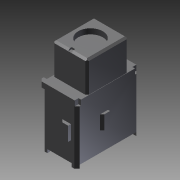
# Autodesk Inventor part: A1-toggle-body
Saved by Autodesk Inventor 2011 SP1 (Build 150282100, 282)
## iProperties
Created: 2013-12-24
Part Number: A1-toggle-body
Catalog Web Link: www.cadenas.de
Description: A Series - Process Sealed Subminiature Toggle -body-
Vendor: NKKSWITCHES
Document SubType Name: Modeling
Designer: PARTuser1
Manufacturer: NKKSWITCHES
Density: 1 g/cm^3
Category: PARTsolutions
Company: NKKSWITCHES
Title: A1-toggle-body
Author: Cadenas PARTsolutions
PSOL_IDENT_0: {$CADENAS_DATA\23d-libs\nkkswitches\toggle\a\parts\a_toggle_body.prj},218 {VTYP=3D},{NB=A1-toggle-bo
PSOL_IDENT_1: dy},{LINA=A1-toggle-body},{NN=A Series - Process Sealed Subminiature Toggle -body},{DATE=12.03.2009
PSOL_IDENT_2: 11:33:35},{GEOMDATE=26.02.2009 12:28:00},{VERSION=},{LINEID=10},{LINESUBID=-1},{WBVAR=PLS}  {NB=A1-t
PSOL_IDENT_3: oggle-body},{LINA=A1-toggle-body},{KT=DUMMY},{PN=A1},{SRS=A},{PLS=1}
CNS_NN: A Series - Process Sealed Subminiature Toggle -body
CNS_NB: A1-toggle-body
CNS_NBSYN: $PN.-toggle-body
CNS_LINA: A1-toggle-body
CNS_PN: A1
CNS_SRS: A
CNS_PLS: 1 - SPDT
SUPPLIER: NKKSWITCHES
ARTICLENO: A1-toggle-body
BOMINFO: A1-toggle-body
CREATOR: CADENAS GmbH
Autodesk Inventor part; units mm, degrees
sketch "Sketch_1" plane through (0, 0, 0) normal (0, 1, 0) x (-1, 0, 0)
  line L0 (2.54, -4.1148) -> (2.54, 4.1148)
  line L1 (2.54, 4.1148) -> (2.159, 4.4958)
  line L2 (2.159, 4.4958) -> (-2.159, 4.4958)
  line L3 (-2.159, 4.4958) -> (-2.54, 4.1148)
  line L4 (-2.54, 4.1148) -> (-2.54, -4.1148)
  line L5 (-2.54, -4.1148) -> (-2.159, -4.4958)
  line L6 (-2.159, -4.4958) -> (2.159, -4.4958)
  line L7 (2.159, -4.4958) -> (2.54, -4.1148)
  constraints: 16 end point
extrude "Extrusion1" add sketch "Sketch_1" against normal blind 8.6106
sketch "Sketch_2" plane through (0, -8.6106, 0) normal (0, 1, 0) x (1, 0, 0)
  line L0 (-2.54, 3.7338) -> (-2.54, -3.7338)
  line L1 (-2.54, -3.7338) -> (-2.159, -3.7338)
  line L2 (-2.159, -3.7338) -> (-2.159, -4.1148)
  line L3 (-2.159, -4.1148) -> (-1.778, -4.1148)
  line L4 (-1.778, -4.1148) -> (-1.778, -4.4958)
  line L5 (-1.778, -4.4958) -> (1.778, -4.4958)
  line L6 (1.778, -4.4958) -> (1.778, -4.1148)
  line L7 (1.778, -4.1148) -> (2.54, -4.1148)
  line L8 (2.54, -4.1148) -> (2.54, 4.1148)
  line L9 (2.54, 4.1148) -> (1.778, 4.1148)
  line L10 (1.778, 4.1148) -> (1.778, 4.4958)
  line L11 (1.778, 4.4958) -> (-1.778, 4.4958)
  line L12 (-1.778, 4.4958) -> (-1.778, 4.1148)
  line L13 (-1.778, 4.1148) -> (-2.159, 4.1148)
  line L14 (-2.159, 4.1148) -> (-2.159, 3.7338)
  line L15 (-2.159, 3.7338) -> (-2.54, 3.7338)
  constraints: 32 end point
extrude "Extrusion2" cut sketch "Sketch_2" along normal blind 0.508
sketch "Sketch_21" plane through (0, -8.6106, 0) normal (0, 1, 0) x (1, 0, 0)
  line L0 (-2.159, -4.1148) -> (2.159, -4.1148)
  line L1 (2.159, -4.1148) -> (2.159, 4.1148)
  line L2 (2.159, 4.1148) -> (-2.159, 4.1148)
  line L3 (-2.159, 4.1148) -> (-2.159, -4.1148)
  constraints: 8 end point
extrude "Extrusion3" cut sketch "Sketch_21" along normal blind 0.9144
sketch "Sketch_3" plane through (0, 0, 0) normal (0, 1, 0) x (-1, 0, 0)
  line L0 (-2.1717, -3.9243) -> (-2.6162, -3.9243)
  line L1 (-2.6162, -3.9243) -> (-2.6162, 3.9243)
  line L2 (-2.6162, 3.9243) -> (-2.1717, 3.9243)
  line L3 (-2.1717, 3.9243) -> (-2.1717, 4.4958)
  line L4 (-2.1717, 4.4958) -> (-2.921, 4.4958)
  line L5 (-2.921, 4.4958) -> (-2.921, -4.4958)
  line L6 (-2.921, -4.4958) -> (-2.1717, -4.4958)
  line L7 (-2.1717, -4.4958) -> (-2.1717, -3.9243)
  constraints: 16 end point
extrude "Extrusion4" cut sketch "Sketch_3" against normal blind 0.762
sketch "Sketch_4" plane through (0, 0, 0) normal (0, 1, 0) x (-1, 0, 0)
  line L0 (2.9972, -3.81) -> (2.5019, -3.81)
  line L1 (2.5019, -3.81) -> (2.5019, 3.81)
  line L2 (2.5019, 3.81) -> (2.9972, 3.81)
  line L3 (2.9972, 3.81) -> (2.9972, 4.1148)
  line L4 (2.9972, 4.1148) -> (2.6162, 4.4958)
  line L5 (2.6162, 4.4958) -> (0.0762, 4.4958)
  line L6 (0.0762, 4.4958) -> (0.0762, -4.4958)
  line L7 (0.0762, -4.4958) -> (2.6162, -4.4958)
  line L8 (2.6162, -4.4958) -> (2.9972, -4.1148)
  line L9 (2.9972, -4.1148) -> (2.9972, -3.81)
  constraints: 20 end point
extrude "Extrusion5" add sketch "Sketch_4" against normal blind 0.762
sketch "Sketch_5" plane through (0, -3.241, 0) normal (0, 1, 0) x (1, 0, 0)
  line L0 (0.41, -4.4958) -> (0.8164, -4.9022)
  line L1 (0.8164, -4.9022) -> (1.651, -4.9022)
  line L2 (1.651, -4.9022) -> (1.651, -4.4958)
  line L3 (1.651, -4.4958) -> (0.41, -4.4958)
  constraints: 8 end point
extrude "Extrusion6" add sketch "Sketch_5" against normal blind 2.032
sketch "Sketch_6" plane through (0, -3.241, 0) normal (0, 1, 0) x (1, 0, 0)
  line L0 (0.41, 4.4958) -> (1.651, 4.4958)
  line L1 (1.651, 4.4958) -> (1.651, 4.9022)
  line L2 (1.651, 4.9022) -> (0.8164, 4.9022)
  line L3 (0.8164, 4.9022) -> (0.41, 4.4958)
  constraints: 8 end point
extrude "Extrusion7" add sketch "Sketch_6" against normal blind 2.032
sketch "Sketch_7" plane through (0, -3.241, 0) normal (0, 1, 0) x (1, 0, 0)
  line L0 (2.54, 0) -> (2.54, -1.1394)
  line L1 (2.54, -1.1394) -> (2.8448, -0.8346)
  line L2 (2.8448, -0.8346) -> (2.8448, 0)
  line L3 (2.8448, 0) -> (2.54, 0)
  constraints: 8 end point
extrude "Extrusion8" add sketch "Sketch_7" against normal blind 2.032
sketch "Sketch_8" plane through (0, 0, 0) normal (0, 1, 0) x (-1, 0, 0)
  line L0 (2.5019, -2.7432) -> (2.5019, 2.7432)
  line L1 (2.5019, 2.7432) -> (2.2479, 2.9972)
  line L2 (2.2479, 2.9972) -> (-2.2479, 2.9972)
  line L3 (-2.2479, 2.9972) -> (-2.5019, 2.7432)
  line L4 (-2.5019, 2.7432) -> (-2.5019, -2.7432)
  line L5 (-2.5019, -2.7432) -> (-2.2479, -2.9972)
  line L6 (-2.2479, -2.9972) -> (2.2479, -2.9972)
  line L7 (2.2479, -2.9972) -> (2.5019, -2.7432)
  constraints: 16 end point
extrude "Extrusion9" add sketch "Sketch_8" along normal blind 4.4958
sketch "Sketch_9" plane through (0, 0, 0) normal (1, 0, 0) x (0, 1, 0)
  line L0 (0, 3.2953) -> (0, 2.9972)
  line L1 (0, 2.9972) -> (4.2418, 2.9972)
  line L2 (4.2418, 2.9972) -> (4.4958, 2.7432)
  line L3 (4.4958, 2.7432) -> (4.4958, -2.7432)
  line L4 (4.4958, -2.7432) -> (4.2418, -2.9972)
  line L5 (4.2418, -2.9972) -> (0, -2.9972)
  line L6 (0, -2.9972) -> (0, -3.2953)
  line L7 (0, -3.2953) -> (4.5957, -3.2953)
  line L8 (4.5957, -3.2953) -> (4.5957, 3.2953)
  line L9 (4.5957, 3.2953) -> (0, 3.2953)
  constraints: 20 end point
extrude "Extrusion10" cut sketch "Sketch_9" along normal mid plane 5.0038
sketch "Sketch_10" plane through (0, 0, 0) normal (0, 0, 1) x (1, 0, 0)
  line L0 (-3.2953, 0) -> (-2.5019, 0)
  line L1 (-2.5019, 0) -> (-2.5019, 4.2418)
  line L2 (-2.5019, 4.2418) -> (-2.2479, 4.4958)
  line L3 (-2.2479, 4.4958) -> (2.2479, 4.4958)
  line L4 (2.2479, 4.4958) -> (2.5019, 4.2418)
  line L5 (2.5019, 4.2418) -> (2.5019, 0)
  line L6 (2.5019, 0) -> (3.2953, 0)
  line L7 (3.2953, 0) -> (3.2953, 4.5957)
  line L8 (3.2953, 4.5957) -> (-3.2953, 4.5957)
  line L9 (-3.2953, 4.5957) -> (-3.2953, 0)
  constraints: 20 end point
extrude "Extrusion11" cut sketch "Sketch_10" along normal mid plane 5.9944
sketch "Sketch12" plane through (0, 4.4958, 0) normal (0, 1, 0) x (1, 0, 0)
  point P0 (0, 0)
hole "Drilling 1" at (0, 4.4958, 0) direction (0, -1, 0) diameter 3.556 depth 0.762
sketch "Sketch_28" plane through (0, 4.4958, 0) normal (0, 1, 0) x (1, 0, 0)
  line L0 (-0.254, -2.4892) -> (-0.254, -2.9972)
  line L1 (-0.254, -2.9972) -> (0.254, -2.9972)
  line L2 (0.254, -2.9972) -> (0.254, -2.4892)
  line L3 (0.254, -2.4892) -> (-0.254, -2.4892)
  constraints: 8 end point
extrude "Extrusion12" cut sketch "Sketch_28" against normal blind 0.254
ref_plane "to_bracket_r_XY" through (-2.54, -4.3078, 0) normal (1, 0, 0) x (0, 0, -1)
ref_plane "to_bracket_r_YZ" through (-2.54, -4.3078, 0) normal (0, 0, -1) x (0, 1, 0)
ref_plane "to_bracket_r_ZX" through (-2.54, -4.3078, 0) normal (0, 1, 0) x (1, 0, 0)
ref_plane "to_bracket_r2_XY" through (-4.3942, -4.318, 0) normal (1, 0, 0) x (0, 0, -1)
ref_plane "to_bracket_r2_YZ" through (-4.3942, -4.318, 0) normal (0, 0, -1) x (0, 1, 0)
ref_plane "to_bracket_r2_ZX" through (-4.3942, -4.318, 0) normal (0, 1, 0) x (1, 0, 0)
ref_plane "to_bracket_s_XY" through (-2.54, -4.7015, 0) normal (1, 0, 0) x (0, 0, -1)
ref_plane "to_bracket_s_YZ" through (-2.54, -4.7015, 0) normal (0, 0, -1) x (0, 1, 0)
ref_plane "to_bracket_s_ZX" through (-2.54, -4.7015, 0) normal (0, 1, 0) x (1, 0, 0)
ref_plane "to_bracket_s2_XY" through (-4.3942, -4.7142, 0) normal (1, 0, 0) x (0, 0, -1)
ref_plane "to_bracket_s2_YZ" through (-4.3942, -4.7142, 0) normal (0, 0, -1) x (0, 1, 0)
ref_plane "to_bracket_s2_ZX" through (-4.3942, -4.7142, 0) normal (0, 1, 0) x (1, 0, 0)
ref_plane "to_bracket_v_XY" through (0, -4.1554, 4.3942) normal (0, 0, -1) x (1, 0, 0)
ref_plane "to_bracket_v_YZ" through (0, -4.1554, 4.3942) normal (1, 0, 0) x (0, -1, 0)
ref_plane "to_bracket_v_ZX" through (0, -4.1554, 4.3942) normal (0, -1, 0) x (0, 0, -1)
ref_plane "to_dummy_XY" through (0, 0, 0) normal (0, -1, 0) x (1, 0, 0)
ref_plane "to_dummy_YZ" through (0, 0, 0) normal (1, 0, 0) x (0, 0, 1)
ref_plane "to_dummy_ZX" through (0, 0, 0) normal (0, 0, 1) x (0, -1, 0)
ref_plane "to_terminal_XY" through (0, -7.3406, 0) normal (0, 1, 0) x (1, 0, 0)
ref_plane "to_terminal_YZ" through (0, -7.3406, 0) normal (1, 0, 0) x (0, 0, -1)
ref_plane "to_terminal_ZX" through (0, -7.3406, 0) normal (0, 0, -1) x (0, 1, 0)
ref_plane "to_toggle_XY" through (0, 4.4958, 0) normal (0, -1, 0) x (1, 0, 0)
ref_plane "to_toggle_YZ" through (0, 4.4958, 0) normal (1, 0, 0) x (0, 0, 1)
ref_plane "to_toggle_ZX" through (0, 4.4958, 0) normal (0, 0, 1) x (0, -1, 0)
body "Solid1"
